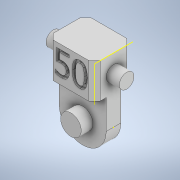
# Autodesk Inventor part: 1번부품
Saved by Autodesk Inventor 2022 (Build 260153000, 153)
## iProperties
Created: 2021-09-05
Part Number: 1번부품
Material: 일반
Document SubType Name: Modeling
Designer: 서울공업고등학교
Density: 1 g/cm^3
Appearance: 기본값
Author: 서울공업고등학교
Autodesk Inventor part; units mm, degrees
ref_plane "YZ Plane" through (0, 0, 0) normal (1, 0, 0) x (0, 1, 0)
ref_plane "XZ Plane" through (0, 0, 0) normal (0, 1, 0) x (-1, 0, 0)
ref_plane "XY Plane" through (0, 0, 0) normal (0, 0, 1) x (1, 0, 0)
sketch "스케치1" plane through (0, 0, 0) normal (0, 0, 1) x (1, 0, 0)
  circle A0 centre (0, 0) radius 3.5
  line L0 (-8, 22) -> (8, 22)
  line L1 (8, 22) -> (8, -8)
  line L2 (8, -8) -> (-8, -8)
  line L3 (-8, -8) -> (-8, 22)
  line L4 (-8, 10) -> (8, 10)
  dimension "d0" = 7
  dimension "d2" = 16
  dimension "d3" = 8
  dimension "d4" = 30
  dimension "d5" = 22
  dimension "d6" = 12
  constraints: 10 end point, 2 horizontal, 2 parallel, 2 point on line, 1 centre point, 1 coincident, 1 perpendicular
  measures "d0" diameter of A0
  measures "d2" distance of L0.start L0.end
  measures "d3" distance from line of point (0, 0) L3
  measures "d4" distance of L0.end L1.end
  measures "d5" distance from line of point (0, 0) L0
  measures "d6" distance between parallel lines of L4 L0
extrude "돌출1" add sketch "스케치1" along normal mid plane 13 contours A0
extrude "돌출2" add sketch "스케치1" along normal mid plane 5 contours L4 L1 L2 L3
extrude "돌출3" add sketch "스케치1" along normal mid plane 13 contours L0 L1 L4 L3
sketch "스케치2" plane through (8, -8, 2.5) normal (1, 0, 0) x (0, 0, -1)
  line L0 (9, 30) -> (-4, 30) projected
  line L1 (-4, 18) -> (-4, 30) projected
  point P0 (2.5, 8)
sketch "스케치3" plane through (0, 0, 0) normal (1, 0, 0) x (0, 1, 0)
  circle A0 centre (16, 0) radius 2.5
  line L0 (22, 6.5) -> (22, -6.5) projected
  line L1 (22, 6.5) -> (10, 6.5) projected
  point P0 (0, 0)
  dimension "d16" = 5
  dimension "d17" = 6
  dimension "d18" = 6.5
  constraints: 1 centre point
  measures "d16" diameter of A0
  measures "d17" distance from line of L0 A0.centre
  measures "d18" distance from line of L1 A0.centre
extrude "돌출4" add sketch "스케치3" along normal mid plane 25
fillet "모깎기1" radius 8 2 edges at (8, -8, 0) (-8, -8, 0)
chamfer "모따기1" distance 2 angle 45 4 edges at (8, 16, 6.5) (8, 16, -6.5) (-8, 16, 6.5) (-8, 16, -6.5)
sketch "스케치4" plane through (0, 0, 6.5) normal (0, 0, 1) x (1, 0, 0)
  line L0 (-5.9498, 20.5659) -> (5.0498, 20.5659) construction
  line L1 (5.0498, 20.5659) -> (5.0498, 12.6328) construction
  line L2 (5.0498, 12.6328) -> (-5.9498, 12.6328) construction
  line L3 (-5.9498, 12.6328) -> (-5.9498, 20.5659) construction
  spline S0 degree 2 poles (-0.517, 14.9451) (-0.517, 14.3681) (-0.8866, 13.3827) (-1.2237, 13.0197) knots 0 0 0 1 2 2 2
  spline S1 degree 2 poles (-1.2237, 13.0197) (-1.5608, 12.6566) (-2.5657, 12.2352) (-3.188, 12.2352) knots 0 0 0 1 2 2 2
  spline S2 degree 2 poles (-3.188, 12.2352) (-3.7585, 12.2352) (-4.8736, 12.4881) (-5.282, 12.689) knots 0 0 0 1 2 2 2
  line L4 (-5.282, 12.689) -> (-5.282, 13.8236)
  line L5 (-5.282, 13.8236) -> (-5.2042, 13.8236)
  spline S3 degree 2 poles (-5.2042, 13.8236) (-5.081, 13.7328) (-4.6208, 13.4994) (-4.342, 13.3957) knots 0 0 0 1 2 2 2
  spline S4 degree 2 poles (-4.342, 13.3957) (-4.0243, 13.2855) (-3.4992, 13.1623) (-3.1686, 13.1623) knots 0 0 0 1 2 2 2
  spline S5 degree 2 poles (-3.1686, 13.1623) (-2.8444, 13.1623) (-2.235, 13.3957) (-2.0146, 13.6485) knots 0 0 0 1 2 2 2
  spline S6 degree 2 poles (-2.0146, 13.6485) (-1.8136, 13.8884) (-1.6062, 14.5237) (-1.6062, 14.9516) knots 0 0 0 1 2 2 2
  spline S7 degree 2 poles (-1.6062, 14.9516) (-1.6062, 15.3795) (-1.8396, 15.9241) (-2.06, 16.1056) knots 0 0 0 1 2 2 2
  spline S8 degree 2 poles (-2.06, 16.1056) (-2.2869, 16.3066) (-2.9611, 16.4751) (-3.3695, 16.4751) knots 0 0 0 1 2 2 2
  spline S9 degree 2 poles (-3.3695, 16.4751) (-3.8104, 16.4751) (-4.6856, 16.339) (-4.9514, 16.2806) knots 0 0 0 1 2 2 2
  line L6 (-4.9514, 16.2806) -> (-4.9514, 20.4038)
  line L7 (-4.9514, 20.4038) -> (-0.5624, 20.4038)
  line L8 (-0.5624, 20.4038) -> (-0.5624, 19.4638)
  line L9 (-0.5624, 19.4638) -> (-3.9206, 19.4638)
  line L10 (-3.9206, 19.4638) -> (-3.9206, 17.3309)
  spline S10 degree 2 poles (-3.9206, 17.3309) (-3.7261, 17.3568) (-3.3501, 17.3762) (-3.1945, 17.3762) knots 0 0 0 1 2 2 2
  spline S11 degree 2 poles (-3.1945, 17.3762) (-2.5786, 17.3762) (-1.7293, 17.1753) (-1.3404, 16.8771) knots 0 0 0 1 2 2 2
  spline S12 degree 2 poles (-1.3404, 16.8771) (-0.9449, 16.5788) (-0.517, 15.6712) (-0.517, 14.9451) knots 0 0 0 1 2 2 2
  spline S13 degree 2 poles (5.6159, 16.4038) (5.6159, 14.2514) (4.3647, 12.2352) (3.0616, 12.2352) knots 0 0 0 1 2 2 2
  spline S14 degree 2 poles (3.0616, 12.2352) (1.739, 12.2352) (0.5008, 14.2903) (0.5008, 16.3973) knots 0 0 0 1 2 2 2
  spline S15 degree 2 poles (0.5008, 16.3973) (0.5008, 18.5626) (1.752, 20.5659) (3.0616, 20.5659) knots 0 0 0 1 2 2 2
  spline S16 degree 2 poles (3.0616, 20.5659) (4.3776, 20.5659) (5.6159, 18.4913) (5.6159, 16.4038) knots 0 0 0 1 2 2 2
  spline S17 degree 2 poles (4.2415, 13.9662) (4.3971, 14.3617) (4.5267, 15.5805) (4.5267, 16.4038) knots 0 0 0 1 2 2 2
  spline S18 degree 2 poles (4.5267, 16.4038) (4.5267, 17.2271) (4.3971, 18.4395) (4.235, 18.8479) knots 0 0 0 1 2 2 2
  spline S19 degree 2 poles (4.235, 18.8479) (4.0729, 19.2563) (3.5089, 19.6777) (3.0616, 19.6777) knots 0 0 0 1 2 2 2
  spline S20 degree 2 poles (3.0616, 19.6777) (2.6143, 19.6777) (2.0373, 19.2563) (1.8687, 18.8349) knots 0 0 0 1 2 2 2
  spline S21 degree 2 poles (1.8687, 18.8349) (1.7066, 18.4265) (1.5899, 17.1818) (1.5899, 16.3973) knots 0 0 0 1 2 2 2
  spline S22 degree 2 poles (1.5899, 16.3973) (1.5899, 15.5545) (1.6937, 14.4265) (1.8622, 13.9856) knots 0 0 0 1 2 2 2
  spline S23 degree 2 poles (1.8622, 13.9856) (2.0178, 13.5707) (2.5948, 13.1234) (3.0616, 13.1234) knots 0 0 0 1 2 2 2
  spline S24 degree 2 poles (3.0616, 13.1234) (3.5024, 13.1234) (4.0794, 13.5448) (4.2415, 13.9662) knots 0 0 0 1 2 2 2
  point P0 (0, 0)
  constraints: 2 other
extrude "돌출5" cut sketch "스케치4" against normal blind 1
